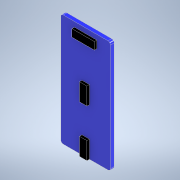
# Autodesk Inventor part: Placa
Saved by Autodesk Inventor 2021 (Build 250183000, 183)
## iProperties
Created: 2021-06-10
Part Number: Placa
Material: Genérico
Document SubType Name: Modeling
Designer: rubia
Density: 1 g/cm^3
Appearance: Liso - Preto
Author: rubia
Autodesk Inventor part; units mm, degrees
ref_plane "YZ Plane" through (0, 0, 0) normal (1, 0, 0) x (0, 1, 0)
ref_plane "XZ Plane" through (0, 0, 0) normal (0, 1, 0) x (-1, 0, 0)
ref_plane "XY Plane" through (0, 0, 0) normal (0, 0, 1) x (1, 0, 0)
sketch "Esboço1" plane through (0, 0, 0) normal (0, 0, 1) x (1, 0, 0)
  line L0 (0, 0) -> (20, 0)
  line L1 (20, 0) -> (20, 45)
  line L2 (20, 45) -> (0, 45)
  line L3 (0, 45) -> (0, 0)
  line L4 (7.3975, 0) -> (10.3975, 0)
  dimension "d0" = 20
  dimension "d1" = 45
  constraints: 10 end point, 2 horizontal, 2 parallel, 1 perpendicular, 1 point on line
  measures "d0" distance of L2.end L1.end
  measures "d1" distance of L1.end L0.end
extrude "Extrusão1" add sketch "Esboço1" along normal blind 1.5
fillet "Arredondamento1" radius 1 4 edges at (20, 45, 0.75) (20, 0, 0.75) (0, 45, 0.75) (0, 0, 0.75)
sketch "Esboço2" plane through (0, 0, 1.5) normal (0, 0, 1) x (1, 0, 0)
  line L0 (1, 0) -> (19, 0) projected
  line L1 (8.5, 0) -> (11.5, 0)
  line L2 (11.5, 0) -> (11.5, 7)
  line L3 (11.5, 7) -> (8.5, 7)
  line L4 (8.5, 7) -> (8.5, 0)
  line L5 (8.5, 19) -> (11.5, 19)
  line L6 (11.5, 19) -> (11.5, 26)
  line L7 (11.5, 26) -> (8.5, 26)
  line L8 (8.5, 26) -> (8.5, 19)
  line L9 (10, 7) -> (10, 0) construction
  line L10 (0, 44) -> (0, 1) construction
  line L11 (11.5, 22.5) -> (8.5, 22.5) construction
  line L12 (19, 45) -> (1, 45) projected
  line L13 (5.5, 43) -> (14.5, 43)
  line L14 (14.5, 43) -> (14.5, 40)
  line L15 (14.5, 40) -> (5.5, 40)
  line L16 (5.5, 40) -> (5.5, 43)
  point P0 (0, 0)
  dimension "d9" = 3
  dimension "d10" = 7
  dimension "d11" = 3
  dimension "d12" = 7
  dimension "d13" = 10
  dimension "d19" = 12
  dimension "d20" = 9
  dimension "d21" = 3
  dimension "d22" = 2
  dimension "d23" = 5.5
  constraints: 28 end point, 6 parallel, 4 midpoint, 3 horizontal, 3 perpendicular, 2 point on line
  measures "d9" distance of L3.end L2.end
  measures "d10" distance of L2.end L1.end
  measures "d11" distance of L7.end L6.end
  measures "d12" distance of L6.end L5.end
  measures "d13" distance between parallel lines of L9 L10
  measures "d19" distance between parallel lines of L5 L3
  measures "d20" distance of L14.end L15.end
  measures "d21" distance of L13.end L14.end
  measures "d22" distance between parallel lines of L12 L13
  measures "d23" distance between parallel lines of L16 L10
extrude "Extrusão2" add sketch "Esboço2" along normal blind 1 separate body
sketch "Esboço3" plane through (0, 0, 0) normal (0, 0, -1) x (-1, 0, 0)
  line L0 (-20, 1) -> (-20, 44) construction
  line L1 (-1, 0) -> (-19, 0) projected
  line L2 (-1.75, 18.25) -> (-1.75, 26.75) construction
  line L3 (-0.5, 19.5) -> (-0.5, 25.5)
  line L4 (-3, 25.5) -> (-3, 19.5)
  arc A0 (-3, 19.5) -> (-0.5, 19.5) centre (-1.75, 19.5) ccw
  arc A1 (-0.5, 25.5) -> (-3, 25.5) centre (-1.75, 25.5) ccw
  line L5 (0, 44) -> (0, 1) projected
  point P0 (0, 0)
  point P1 (-8.5, 19)
  point P2 (-8.5, 26)
  point P3 (-1.75, 22.5)
  dimension "d30" = 8.5
  dimension "d31" = 2.5
  dimension "d32" = 22.5
  dimension "d33" = 6
  dimension "d34" = 1.25
  dimension "d35" = 0.5
  constraints: 8 end point, 6 point on circle, 4 tangent, 2 centre point, 2 point on line, 1 midpoint, 1 parallel, 1 vertical
  measures "d30" distance of L2.start L2.end
  measures "d31" diameter of A1
  measures "d32" distance from line of L1 point (-1.75, 22.5)
  measures "d33" distance of A1.centre A0.centre
  measures "d34" radius of A1
  measures "d35" distance between parallel lines of L5 L3
extrude "Extrusão3" add sketch "Esboço3" along normal blind 3 bodies 1
